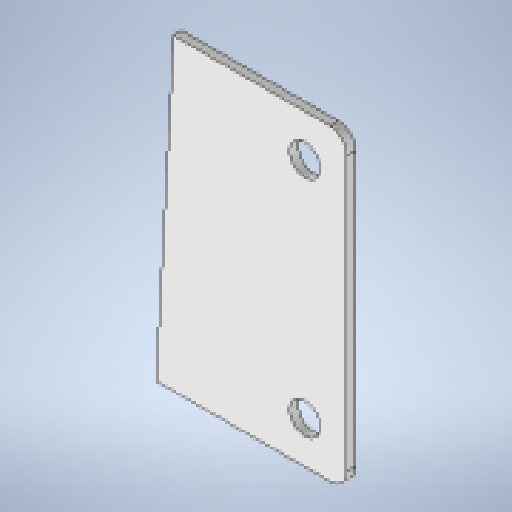
# Autodesk Inventor part: MSC 815 wall inner joint
Saved by Autodesk Inventor 2025 (Build 290162010, 162A)
## iProperties
Created: 2024-04-18
Part Number: MSC 815 wall inner joint
Material: AISI304
Document SubType Name: Sheet Metal
Designer: admin
Stock Number: МОО 813 стойка боковая жабры
Mass: 2919.69 g
Surface Area: 2571.84 cm^2
Volume: 364.962 cm^3
Density: 8 g/cm^3
Flat Pattern Width: 6.8 cm
Flat Pattern Length: 11 cm
Flat Pattern Area: 74.8 cm^2
Sheet Metal Rule: AISI304 3mm
Sheet Metal Width: 68,000 mm
Sheet Metal Length: 110,000 mm
Sheet Metal Area: 7480,000 mm^2
Appearance: Default
Author: admin
Autodesk Inventor part; units mm, degrees
ref_plane "YZ Plane" through (0, 0, 0) normal (1, 0, 0) x (0, 1, 0)
ref_plane "XZ Plane" through (0, 0, 0) normal (0, 1, 0) x (-1, 0, 0)
ref_plane "XY Plane" through (0, 0, 0) normal (0, 0, 1) x (1, 0, 0)
sketch "Sketch1" plane through (0, 0, 0) normal (0, 0, 1) x (1, 0, 0)
  line L0 (-34, 55) -> (34, 55)
  line L1 (34, 55) -> (34, -55)
  line L2 (34, -55) -> (-34, -55)
  line L3 (-34, -55) -> (-34, 55)
  line L4 (-34, 55) -> (34, -55) construction
  line L5 (34, 55) -> (-34, -55) construction
  line L6 (-34, -19) -> (-34, 19)
  circle A0 centre (19, 40) radius 5.5
  circle A1 centre (19, -40) radius 5.5
  line L7 (0, 0) -> (34, 0) construction
  line L8 (-34, -55) -> (-28, 55)
  dimension "d157" = 68
  dimension "d158" = 110
  dimension "d160" = 80
  dimension "d161" = 11
  dimension "d164" = 15
  dimension "d165" = 6
  measures "d157" distance of L0.start L0.end
  measures "d158" distance of L0.end L1.end
  measures "d160" distance of A1.centre A0.centre
  measures "d161" diameter of A0
  measures "d164" distance from line of A0.centre L1
  measures "d165" distance of L0.start L8.end
extrude "Plate3" add sketch "Sketch1" along normal blind 3 contours L0 L1 L2 L8
fillet "Corner Round2" radius 6 2 edges at (34, 55, 1.5) (34, -55, 1.5)
equation "\"BendReliefWidth\" = Thickness"
equation "\"BendReliefDepth\" = 0.5 * Thickness"
equation "\"CornerReliefSize\" = 4 * Thickness"
equation "\"MinimumRemnant\" = 2 * Thickness"
equation "\"GapSize\" = Thickness"
equation "\"Thickness\" = 3"
body "Solid4"
